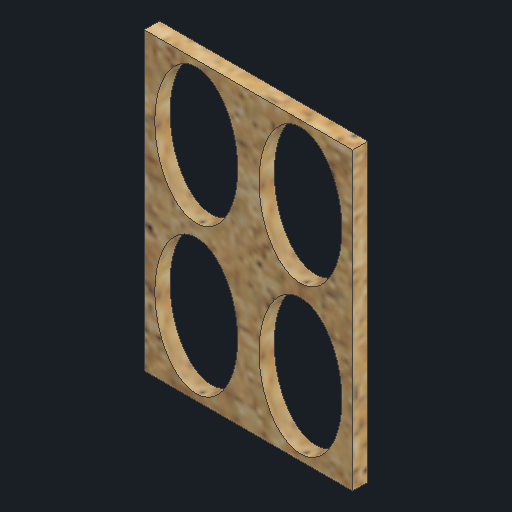
# Autodesk Inventor part: ArmDesk
Saved by Autodesk Inventor 2022 (Build 260153070, 153G)
## iProperties
Created: 2021-12-13
Part Number: ArmDesk
Material: Древесно-стружечная плита
Document SubType Name: Modeling
Designer: A
Density: 0.8 g/cm^3
Appearance: Древесно-стружечная плита
Mass: 369.649 g
Surface Area: 978.831 cm^2
Volume: 462.062 cm^3
Author: A
Autodesk Inventor part; units mm, degrees
ref_plane "YZ Plane" through (0, 0, 0) normal (1, 0, 0) x (0, 1, 0)
ref_plane "XZ Plane" through (0, 0, 0) normal (0, 1, 0) x (-1, 0, 0)
ref_plane "XY Plane" through (0, 0, 0) normal (0, 0, 1) x (1, 0, 0)
sketch "Эскиз1" plane through (0, 0, 0) normal (0, 0, 1) x (1, 0, 0)
  line L0 (0, 0) -> (218, 0)
  line L1 (218, 0) -> (218, -309)
  line L2 (218, -309) -> (0, -309)
  line L3 (0, -309) -> (0, 0)
  line L4 (0, 0) -> (218, -309)
  line L5 (218, 0) -> (0, -309) construction
  line L6 (0, -154.5) -> (218, -154.5) construction
  line L7 (109, 0) -> (109, -309) construction
  line L8 (109, 0) -> (0, -154.5) construction
  line L9 (0, -154.5) -> (109, -309) construction
  line L10 (109, -309) -> (218, -154.5) construction
  line L11 (218, -154.5) -> (109, 0) construction
  ellipse E0 centre (163.5, -231.75) end of major axis (163.5, -161.0034) minor radius 43.2868
  ellipse E1 centre (54.5, -231.75) end of major axis (54.5, -161.0034) minor radius 43.2868
  ellipse E2 centre (163.5, -77.25) end of major axis (163.5, -6.5034) minor radius 43.2868
  ellipse E3 centre (54.5, -77.25) end of major axis (54.5, -6.5034) minor radius 43.2868
  dimension "d0" = 218
  dimension "d1" = 309
  constraints: 24 end point, 9 midpoint, 4 parallel, 2 point on line, 1 horizontal, 8 other
  measures "d0" distance of L1.end L2.end
  measures "d1" distance of L0.end L1.end
extrude "Выдавливание2" add sketch "Эскиз1" along normal blind 16 contours L4 E3 E0 L2 L3 | L0 L1 L4 E0 E3
